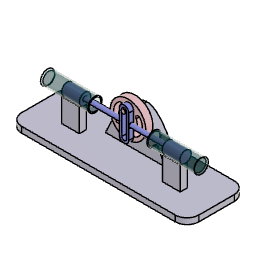
Scotch Yoke Mechanism (Autodesk Fusion 360 design; units mm, degrees)
Autodesk Fusion 360 part; units mm, degrees
note: some values were not read from the file. Set by a fixed rule: which face or edge a step refers to.
sketch "Base" plane through (0, 0, 0) normal (0, 0, 1) x (1, 0, 0) in component "Base"
  line L0 (65, 25) -> (-65, 25)
  line L1 (-75, 15) -> (-75, -15)
  line L2 (-65, -25) -> (65, -25)
  line L3 (75, -15) -> (75, 15)
  arc A0 (-65, 25) -> (-75, 15) centre (-65, 15) ccw
  arc A1 (-75, -15) -> (-65, -25) centre (-65, -15) ccw
  arc A2 (65, -25) -> (75, -15) centre (65, -15) ccw
  arc A3 (75, 15) -> (65, 25) centre (65, 15) ccw
  dimension "d4" = 10
  dimension "d5" = 10
  constraint horizontal L0
  constraint perpendicular L0 L1
  constraint parallel L0 L2
  constraint parallel L1 L3
  constraint tangent L1 A0
  constraint tangent L0 A0
  constraint tangent L2 A1
  constraint tangent L1 A1
  constraint equal A0 A1
  constraint tangent L3 A2
  constraint tangent L2 A2
  constraint equal A0 A2
  constraint tangent L0 A3
  constraint tangent L3 A3
  measures "d4" radius of A0
  measures "d5" radius of A3
extrude "Extrude2" add sketch "Base" along normal blind 5 makes body 1 in component "Base"
sketch "Horizontal plane" plane through (0, 0, 5) normal (0, 0, 1) x (-1, 0, 0) in component "Holder"
  arc A0 (-75, -15) -> (-65, -25) centre (-65, -15) ccw
  line L0 (-65, -25) -> (65, -25)
  arc A1 (65, -25) -> (75, -15) centre (65, -15) ccw
  line L1 (75, -15) -> (75, 15)
  arc A2 (75, 15) -> (65, 25) centre (65, 15) ccw
  line L2 (65, 25) -> (-65, 25)
  arc A3 (-65, 25) -> (-75, 15) centre (-65, 15) ccw
  line L3 (-75, 15) -> (-75, -15)
  line L4 (25, -6) -> (-25, -6)
  line L5 (-25, -6) -> (-25, -16)
  line L6 (-25, -16) -> (25, -16)
  line L7 (25, -16) -> (25, -6)
  line L8 (0, -11) -> (0, 25)
  point P0 (0, -11)
  dimension "d8" = 50
  dimension "d9" = 10
  constraint horizontal L4
  constraint perpendicular L4 L5
  constraint parallel L4 L6
  constraint parallel L5 L7
  constraint coincident P0 L8.start
  constraint perpendicular L4 L8
  measures "d8" distance of L5.end L6.end
  measures "d9" distance of L4.end L5.end
extrude "Extrude3" cut sketch "Horizontal plane" against normal blind 5 contours L4 L5 L6 L7 bodies 1 in component "Base"
extrude "Extrude1" add sketch "Horizontal plane" along normal blind 30 and the other way blind 5 separate body contours L4 L5 L6 L7 makes body 2 in component "Holder"
sketch "Vertical plane" plane through (0, 6, 0) normal (0, -1, 0) x (1, 0, 0) in component "Holder"
  line L0 (25, 0) -> (25, 35)
  line L1 (25, 35) -> (-25, 35)
  line L2 (-25, 35) -> (-25, 0)
  line L3 (-25, 0) -> (25, 0)
  spline S0 degree 5 poles (-25, 5) (-24, 7.2754) (-22, 11.6276) (-19, 17.5597) (-15, 24.2571) (-10, 30.4718) (-5, 34.3367) (0, 35.6598) (5, 34.3367) (10, 30.4718) (15, 24.2571) (19, 17.5597) (22, 11.6276) (24, 7.2754) (25, 5) knots 0 0 0 0 0 0 0.1 0.2 0.3 0.4 0.5 0.6 0.7 0.8 0.9 1 1 1 1 1 1
  circle A0 centre (0, 30) radius 1.8
  circle A1 centre (0, 30) radius 4
  line L4 (-25, 5) -> (25, 5)
  point P0 (0, 35)
  constraint coincident L2 S0.start
  constraint coincident L0 S0.end
  constraint concentric A0 A1
  constraint perpendicular L2 L4
extrude "Extrude2'" cut sketch "Vertical plane" against normal blind 40 contours L0 L1 S0 | L1 L2 S0 bodies 2 in component "Holder"
extrude "Extrude3'" add sketch "Vertical plane" along normal blind 6 contours A0 bodies 2 in component "Holder"
sketch "Crank" plane through (0, 6, 0) normal (0, -1, 0) x (1, 0, 0) in component "Crank"
  circle A0 centre (0, 30) radius 15
  circle A1 centre (0, 40) radius 1.8
  line L0 (-5.5, 36.4952) -> (-5, 36.4952) construction
  arc A2 (-5.9881, 35.1859) -> (-5.9881, 24.8141) centre (0, 30) ccw
  arc A3 (-8.9147, 37.9089) -> (-8.9147, 22.0911) centre (-1, 30) ccw
  arc A4 (-5.9881, 35.1859) -> (-8.9147, 37.9089) centre (-7.5, 36.4952) ccw
  arc A5 (-8.9147, 22.0911) -> (-5.9881, 24.8141) centre (-7.5, 23.5048) ccw
  arc A6 (8.9147, 22.0911) -> (8.9147, 37.9089) centre (1, 30) ccw
  arc A7 (5.9881, 24.8141) -> (5.9881, 35.1859) centre (0, 30) ccw
  arc A8 (8.9147, 37.9089) -> (5.9881, 35.1859) centre (7.5, 36.4952) ccw
  arc A9 (5.9881, 24.8141) -> (8.9147, 22.0911) centre (7.5, 23.5048) ccw
  circle A10 centre (0, 30) radius 2
  constraint tangent A2 A4
  constraint tangent A3 A5
  constraint coincident L0.start A4
  constraint concentric A0 A10
extrude "Extrude1'" add sketch "Crank" along normal blind 6 separate body contours A0 | A10 makes body 3 in component "Crank"
extrude "Extrude2''" add sketch "Crank" along normal blind 12 contours A1 bodies 3 in component "Crank"
sketch "Sliding yoke" plane through (0, 0, 0) normal (0, -1, 0) x (1, 0, 0) in component "Piston & sliding yoke"
  circle A0 centre (0, 40) radius 1.8
  arc A1 (5.9881, 24.8141) -> (8.9147, 22.0911) centre (7.5, 23.5048) ccw
  arc A2 (5.9881, 24.8141) -> (5.9881, 35.1859) centre (0, 30) ccw
  arc A3 (8.9147, 37.9089) -> (5.9881, 35.1859) centre (7.5, 36.4952) ccw
  arc A4 (8.9147, 22.0911) -> (8.9147, 37.9089) centre (1, 30) ccw
  arc A5 (-5.9881, 35.1859) -> (-8.9147, 37.9089) centre (-7.5, 36.4952) ccw
  arc A6 (-5.9881, 35.1859) -> (-5.9881, 24.8141) centre (0, 30) ccw
  arc A7 (-8.9147, 22.0911) -> (-5.9881, 24.8141) centre (-7.5, 23.5048) ccw
  arc A8 (-8.9147, 37.9089) -> (-8.9147, 22.0911) centre (-1, 30) ccw
  circle A9 centre (0, 30) radius 15
  line L0 (-4, 40) -> (-4, 20)
  line L1 (4, 40) -> (4, 20)
  arc A10 (-4, 20) -> (4, 20) centre (0, 20) ccw
  arc A11 (4, 40) -> (-4, 40) centre (0, 40) ccw
  line L2 (-35, 28) -> (-35, 32)
  line L3 (35, 32) -> (35, 28)
  line L4 (-35, 32) -> (-4, 32)
  line L5 (4, 32) -> (35, 32)
  line L6 (35, 28) -> (4, 28)
  line L7 (-4, 28) -> (-35, 28)
  line L8 (-2, 39.9886) -> (-1.8857, 19.9892)
  line L9 (2, 40.0114) -> (2.1143, 20.0121)
  arc A12 (2, 40.0114) -> (-2, 39.9886) centre (0, 40) ccw
  arc A13 (-1.8857, 19.9892) -> (2.1143, 20.0121) centre (0.1143, 20.0007) ccw
  point P0 (0, 30)
  dimension "d33" = 70
  constraint tangent L0 A11
  constraint tangent L0 A10
  constraint tangent L1 A11
  constraint tangent L1 A10
  constraint horizontal L6
  constraint perpendicular L2 L6
  constraint parallel L4 L6
  constraint parallel L2 L3
  constraint coincident P0 A2.centre
  constraint coincident L0 L4.end
  constraint collinear L4 L5
  constraint coincident L0 L7.start
  constraint collinear L6 L7
  constraint coincident L1 L5.start
  constraint coincident L1 L6.end
  constraint concentric A11 A12
  constraint tangent L8 A12
  constraint tangent L9 A12
  constraint tangent L8 A13
  constraint tangent L9 A13
  measures "d33" distance of L2.end L3.start
extrude "Extrude3''" add sketch "Sliding yoke" along normal blind 5 and the other way blind -1 separate body contours L0 L1 A10 A11 makes body 4 in component "Piston & sliding yoke"
extrude "Extrude4" add sketch "Sliding yoke" along normal blind 5 and the other way blind -1 contours A2 L1 L5 L6 | A2 A4 L5 L6 | A4 A9 L5 L6 | A9 L3 L5 L6 | A9 L2 L4 L7 | A8 A9 L4 L7 | A6 A8 L4 L7 | A6 L0 L4 L7 bodies 4 in component "Piston & sliding yoke"
fillet "Fillet3" radius 2 8 edges at (-19.5, -5, 32) (-19.5, -5, 28) (19.5, -5, 32) (19.5, -5, 28) (19.5, -1, 32) (19.5, -1, 28) (-19.5, -1, 32) (-19.5, -1, 28) on bodies 4 in component "Piston & sliding yoke"
sketch "Piston" plane through (-35, 0, 0) normal (-1, 0, 0) x (0, -1, 0) in component "Piston & sliding yoke"
  arc A0 (1, 30) -> (5, 30) centre (3, 30) ccw
  arc A1 (5, 30) -> (1, 30) centre (3, 30) ccw
  circle A2 centre (3, 30) radius 5
  dimension "d54" = 10
  constraint concentric A0 A2
  measures "d54" diameter of A2
extrude "Extrude5" add sketch "Piston" along normal blind 15 contours A0 A1 | A2 bodies 4 in component "Piston & sliding yoke"
extrude "Extrude6" add sketch "Piston" along normal blind -85 and the other way blind 70 contours A0 A1 | A2 bodies 4 in component "Piston & sliding yoke"
sketch "Cylinder1" plane through (-35, 0, 0) normal (-1, 0, 0) x (0, -1, 0) in component "Cylinder"
  circle A0 centre (3, 30) radius 5
  circle A1 centre (3, 30) radius 6
  circle A2 centre (3, 30) radius 2
  constraint concentric A0 A1
  constraint concentric A0 A2
extrude "Extrude5'" add sketch "Cylinder1" along normal blind 30 separate body contours A1 makes body 5 in component "Cylinder"
extrude "Extrude6'" add sketch "Cylinder1" along normal blind 30 and the other way blind -29 contours A0 | A2 bodies 5 in component "Cylinder"
sketch "Cylinder2" plane through (35, 0, 0) normal (-1, 0, 0) x (0, -1, 0) in component "Cylinder"
  circle A0 centre (3, 30) radius 5
  arc A1 (1, 30) -> (5, 30) centre (3, 30) ccw
  arc A2 (5, 30) -> (1, 30) centre (3, 30) ccw
  circle A3 centre (3, 30) radius 5
  circle A4 centre (3, 30) radius 2
  circle A5 centre (3, 30) radius 6
  constraint concentric A2 A3
  constraint tangent A0 A3
  constraint concentric A3 A4
  constraint concentric A3 A5
extrude "Extrude7" add sketch "Cylinder2" against normal blind 30 separate body contours A5 makes body 6 in component "Cylinder"
extrude "Extrude8" add sketch "Cylinder2" along normal blind -30 and the other way blind 29 contours A0 A3 | A1 A2 A4 bodies 6 in component "Cylinder"
sketch "Cylinder holder" plane through (0, 0, 5) normal (0, 0, 1) x (-1, 0, 0) in component "Base"
  line L0 (-25, -6) -> (25, -6)
  line L1 (25, -6) -> (25, -16)
  line L2 (25, -16) -> (-25, -16)
  line L3 (-25, -16) -> (-25, -6)
  arc A0 (-75, -15) -> (-65, -25) centre (-65, -15) ccw
  line L4 (-65, -25) -> (65, -25)
  arc A1 (65, -25) -> (75, -15) centre (65, -15) ccw
  line L5 (75, -15) -> (75, 15)
  arc A2 (75, 15) -> (65, 25) centre (65, 15) ccw
  line L6 (65, 25) -> (-65, 25)
  arc A3 (-65, 25) -> (-75, 15) centre (-65, 15) ccw
  line L7 (-75, 15) -> (-75, -15)
  line L8 (50.2, 0) -> (35.2, 0)
  line L9 (35.2, 0) -> (35.2, 6)
  line L10 (35.2, 6) -> (50.2, 6)
  line L11 (50.2, 6) -> (50.2, 0)
  line L12 (0, 5) -> (0, 25)
  line L13 (-35.2, 0) -> (-35.2, 6)
  line L14 (-35.2, 6) -> (-50.2, 6)
  line L15 (-50.2, 6) -> (-50.2, 0)
  line L16 (-50.2, 0) -> (-35.2, 0)
  dimension "d117" = 15
  constraint horizontal L8
  constraint vertical L9
  constraint horizontal L10
  constraint vertical L11
  constraint midpoint L6 L12.end
  constraint perpendicular L6 L12
  constraint symmetric L8.start L12 L15.end
  constraint symmetric L8.end L12 L13.start
  constraint symmetric L9.end L12 L13.end
  constraint symmetric L10.end L12 L14.end
  measures "d117" distance of L8.start L8.end
move_face "OffsetFaces1" offset -0.2 1 faces at (-45, -7.9752, 29.5022) on bodies 4 in component "Piston & sliding yoke"
move_face "OffsetFaces2" offset -0.2 1 faces at (45, -7.9752, 29.5022) on bodies 4 in component "Piston & sliding yoke"
extrude "Extrude9" add 1 faces at (-35, -8.6257, 29.4535) along direction (1, 0, 0) blind 10 on bodies 5 bodies 5 in component "Cylinder"
extrude "Extrude10" add 1 faces at (35, -0.6604, 35.1453) along direction (-1, 0, 0) blind 10 on bodies 6 bodies 6 in component "Cylinder"
extrude "Extrude6''" add sketch "Cylinder holder" along normal up to surface contours L8 L9 L10 L11 end surface at (-38.3333, -8.9925, 29.7009) on bodies 5 bodies 1 in component "Base"
extrude "Extrude7'" add sketch "Cylinder holder" along normal up to surface contours L13 L14 L15 L16 end surface at (55, -8.9702, 29.4026) on bodies 6 bodies 1 in component "Base"
extrude "Extrude3'''" cut 1 faces at (-0.1335, 0, 30.585) along direction (0, 1, 0) blind 16 on bodies 2 bodies 3 in component "Crank"
component "Crank" placed x (0, 0, 1) y (0, 1, 0) z (-1, 0, 0) at (30, 0, 30)
component "Holder" placed x (1, 0, 0) y (0, 1, 0) z (0, 0, 1) at (0, 0, 0)
component "Base" placed x (1, 0, 0) y (0, 1, 0) z (0, 0, 1) at (0, 0, 0)
component "Piston & sliding yoke" placed x (1, 0, 0) y (0, 1, 0) z (0, 0, 1) at (-10.0573, 0, 0)
component "Cylinder" placed x (1, 0, 0) y (0, 1, 0) z (0, 0, 1) at (0, 0, 0)
named bodies: "Base", "Holder", "Crank", "Piston and sliding yoke", "Cylinder1", "Cylinder2"
